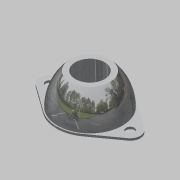
# Autodesk Inventor part: caster_wheel_v5_base
Saved by Autodesk Inventor 2019.3 (Build 233278000, 278)
## iProperties
Created: 2019-03-27
Part Number: caster_wheel_v5_base
Material: Generic
Document SubType Name: Modeling
Designer: Varga Daniel
Density: 1 g/cm^3
Appearance: Aluminum - Dark
Author: Varga Daniel
Autodesk Inventor part; units mm, degrees
ref_plane "YZ Plane" through (0, 0, 0) normal (1, 0, 0) x (0, 1, 0)
ref_plane "XZ Plane" through (0, 0, 0) normal (0, 1, 0) x (-1, 0, 0)
ref_plane "XY Plane" through (0, 0, 0) normal (0, 0, 1) x (1, 0, 0)
sketch "Sketch1" plane through (0, 0, 0) normal (0, 1, 0) x (-1, 0, 0)
  circle A0 centre (19.25, 0) radius 2
  line L0 (0, 16) -> (0, -26.1596) construction
  arc A1 (22.026, -3.8544) -> (22.026, 3.8544) centre (19.25, 0) ccw
  line L1 (22.026, -3.8544) -> (9.3506, -12.9833)
  line L2 (22.026, 3.8544) -> (9.3506, 12.9833)
  line L3 (0, 0) -> (7.2695, 0) construction
  circle A2 centre (-19.25, 0) radius 2
  arc A3 (-22.026, 3.8544) -> (-22.026, -3.8544) centre (-19.25, 0) ccw
  line L4 (-22.026, -3.8544) -> (-9.3506, -12.9833)
  line L5 (-22.026, 3.8544) -> (-9.3506, 12.9833)
  arc A4 (9.3506, 12.9833) -> (-9.3506, 12.9833) centre (0, 0) ccw
  arc A5 (-9.3506, -12.9833) -> (9.3506, -12.9833) centre (0, 0) ccw
  point P0 (-7.2695, 0)
  dimension "d1" = 4
  dimension "d3" = 38.5
  dimension "d6" = 48
  dimension "d9" = 16
  dimension "d10" = 16
  constraints: 12 end point, 9 point on circle, 7 symmetric about line, 6 centre point, 4 tangent, 3 coincident, 2 point on line, 1 perpendicular, 1 vertical, 2 other
  measures "d1" diameter of A0
  measures "d3" diameter of A0.centre L0
  measures "d9" radius of A5
  measures "d10" radius of A4
extrude "Extrusion1" add sketch "Sketch1" along normal blind 1
sketch "Sketch3" plane through (0, 0, 0) normal (0, 0, 1) x (1, 0, 0)
  line L0 (-17.25, 0) -> (-17.25, 1) projected
  line L1 (-17.25, 1) -> (17.25, 1) projected
  line L2 (17.25, 1) -> (17.25, 0) projected
  line L3 (17.25, 0) -> (-17.25, 0) projected
  line L4 (24, 1) -> (24, 0) projected
  line L5 (24, 0) -> (21.25, 0) projected
  line L6 (21.25, 0) -> (21.25, 1) projected
  line L7 (21.25, 1) -> (24, 1) projected
  line L8 (-24, 0) -> (-24, 1) projected
  line L9 (-24, 1) -> (-21.25, 1) projected
  line L10 (-21.25, 1) -> (-21.25, 0) projected
  line L11 (-21.25, 0) -> (-24, 0) projected
  line L12 (0, 1) -> (0, 13.5844) construction
  line L13 (9.3506, 1) -> (-9.3506, 1) projected
  arc A0 (-9.5, 16) -> (-15.5, 1) centre (6.25, 1) ccw
  line L14 (-9.5, 16) -> (-7, 16)
  line L15 (-7, 16) -> (-7, 1)
  line L16 (-7, 1) -> (-15.5, 1)
  line L17 (-22.026, 1) -> (-9.3506, 1) projected
  point P0 (0, 0)
  dimension "d11" = 31
  dimension "d12" = 16
  dimension "d13" = 19
  dimension "d14" = 14
  constraints: 8 end point, 2 point on circle, 2 point on line, 1 centre point, 1 collinear, 1 line through centre, 1 midpoint, 1 parallel, 1 perpendicular, 1 vertical
  measures "d11" diameter of L16.end L12
  measures "d12" distance from line of L14.start L3
  measures "d13" diameter of L14.start L12
  measures "d14" diameter of L14.end L12
revolve "Revolution1" add sketch "Sketch3" angle 360 about axis through (0, 1, 0) along (0, 1, 0) contours A0 L14 L15 L1
equation "\"d10\" = d9"
body "Solid1"
